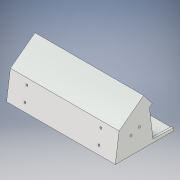
# Autodesk Inventor part: plowV4
Saved by Autodesk Inventor 2019 (Build 230136000, 136)
## iProperties
Created: 2019-04-14
Part Number: plowV4
Material: Generic
Document SubType Name: Modeling
Designer: Tesler
Density: 1 g/cm^3
Appearance: Default
Author: Tesler
Autodesk Inventor part; units mm, degrees
ref_plane "YZ Plane" through (0, 0, 0) normal (1, 0, 0) x (0, 1, 0)
ref_plane "XZ Plane" through (0, 0, 0) normal (0, 1, 0) x (-1, 0, 0)
sketch "Sketch1" plane through (0, 0, 0) normal (1, 0, 0) x (0, 1, 0)
  line L0 (0, 0) -> (0, -85)
  line L1 (0, 0) -> (39.6107, -5.5669)
  line L2 (0, 0) -> (40, 0) construction
  line L3 (39.6107, -5.5669) -> (66.6924, -41.5055)
  line L4 (66.6924, -41.5055) -> (49.9211, -54.1436)
  line L5 (49.9211, -54.1436) -> (47.2715, -49.9034)
  line L6 (0, -85) -> (4, -85)
  line L7 (5, -55) -> (4, -85)
  line L8 (5, -55) -> (47.2715, -49.9034)
  dimension "d0" = 85
  dimension "d1" = 40
  dimension "d2" = 8
  dimension "d3" = 45
  dimension "d4" = 135
  dimension "d5" = 21
  dimension "d6" = 5
  dimension "d7" = 85
  dimension "d12" = 4
  dimension "d13" = 5
  dimension "d50" = 30
  constraints: 18 end point, 2 horizontal, 1 equal length, 1 perpendicular, 1 vertical
  measures "d0" distance of L0.start L0.end
  measures "d1" distance of L0.start L1.end
  measures "d2" angle of L1 L2
  measures "d3" distance of L1.end L3.end
  measures "d4" angle of L1 L3
  measures "d5" distance of L3.end L4.end
  measures "d6" distance of L4.end L5.end
  measures "d7" angle of L4 L5
  measures "d12" distance of L0.end L6.end
  measures "d13" distance from line of L7.start L0
  measures "d50" vertical distance of L7.start L6.end
extrude "Extrusion1" add sketch "Sketch1" along normal blind 3
sketch "Sketch2" plane through (3, 0, 0) normal (1, 0, 0) x (0, 0, -1)
  line L0 (0, 0) -> (85, 0) projected
  line L1 (85, 0) -> (85, 4) projected
  line L2 (85, 4) -> (55, 5) projected
  line L3 (49.9034, 47.2715) -> (54.1436, 49.9211) projected
  line L4 (54.1436, 49.9211) -> (41.5055, 66.6924) projected
  line L5 (41.5055, 66.6924) -> (5.5669, 39.6107) projected
  line L6 (5.5669, 39.6107) -> (0, 0) projected
  line L7 (49.9034, 47.2715) -> (54.1436, 49.9211) projected
  line L8 (51.1436, 48.0464) -> (40.9151, 62.491)
  line L9 (41.5055, 66.6924) -> (5.5669, 39.6107) projected
  line L10 (54.1436, 49.9211) -> (41.5055, 66.6924) projected
  line L11 (40.9151, 62.491) -> (8.3648, 37.9627)
  line L12 (8.3648, 37.9627) -> (3, 3)
  line L13 (5.5669, 39.6107) -> (0, 0) projected
  line L14 (3, 3) -> (85, 3)
  line L15 (85, 0) -> (85, 4) projected
  line L16 (85, 3) -> (85, 0)
  line L17 (0, 0) -> (85, 0) projected
  line L18 (85, 0) -> (0, 0)
  line L19 (0, 0) -> (5.5669, 39.6107)
  line L20 (5.5669, 39.6107) -> (41.5055, 66.6924)
  line L21 (41.5055, 66.6924) -> (54.1436, 49.9211)
  line L22 (54.1436, 49.9211) -> (51.1436, 48.0464)
  line L23 (55, 5) -> (49.9034, 47.2715) projected
  dimension "d14" = 3
  dimension "d15" = 3
  dimension "d16" = 3
  dimension "d17" = 3
  dimension "d18" = 3
  dimension "d21" = 3
  dimension "d22" = 3
  dimension "d23" = 3
  constraints: 20 end point, 4 collinear, 2 point on line, 1 other
  measures "d14" distance from line of L4 L8.end
  measures "d15" horizontal distance of L3.end L8.start
  measures "d16" distance from line of L8.end L5
  measures "d17" distance from line of L5 L11.end
  measures "d18" distance from line of L11.end L6
  measures "d21" distance from line of L0 L14.end
  measures "d22" distance from line of L12.end L0
  measures "d23" horizontal distance of L17.start L12.end
extrude "Extrusion2" add sketch "Sketch2" along normal blind 153 contours L6 L5 L4 L3 L8 L11 L12 L14 L1 L0
ref_plane "Work Plane1" through (79.5, 0, 0) normal (1, 0, 0) x (0, 0, -1)
mirror "Mirror1" about plane through (79.5, 0, 0) normal (1, 0, 0) of "Extrusion1"
sketch "Sketch3" plane through (159, 0, -85) normal (1, 0, 0) x (0, 0, -1)
  line L0 (-85, 0) -> (0, 0) projected
  line L1 (-79.4331, 39.6107) -> (-85, 0) projected
  circle A0 centre (-62.193, 25.4) radius 1.5
  circle A1 centre (-49.984, 30) radius 1.5
  dimension "d28" = 25.4
  dimension "d29" = 30
  dimension "d31" = 19.05
  dimension "d32" = 30.5
  dimension "d33" = 3
  dimension "d34" = 3
  constraints: 2 centre point, 2 coincident
  measures "d28" distance from line of L0 point (-62.193, 25.4)
  measures "d29" distance from line of L0 point (-49.984, 30)
  measures "d31" distance from line of point (-62.193, 25.4) L1
  measures "d32" distance from line of point (-49.984, 30) L1
  measures "d33" diameter of A0
  measures "d34" diameter of A1
extrude "Extrusion3" cut sketch "Sketch3" against normal blind 200
sketch "Sketch4" plane through (0, 0, 0) normal (0, 0.1392, 0.9903) x (1, 0, 0)
  line L0 (0, 0) -> (159, 0) projected
  line L1 (0, 40) -> (0, 0) projected
  line L2 (159, 40) -> (159, 0) projected
  circle A0 centre (25.4, 31.75) radius 1.5
  circle A1 centre (25.4, 11.1125) radius 1.5
  circle A2 centre (133.6, 31.75) radius 1.5
  circle A3 centre (133.6, 11.1125) radius 1.5
  dimension "d37" = 11.1125
  dimension "d38" = 31.75
  dimension "d39" = 25.4
  dimension "d40" = 31.75
  dimension "d41" = 11.1125
  dimension "d42" = 25.4
  dimension "d43" = 3
  dimension "d44" = 3
  dimension "d45" = 3
  dimension "d46" = 3
  constraints: 4 centre point, 4 coincident, 2 vertical alignment
  measures "d37" distance from line of L0 point (25.4, 11.113)
  measures "d38" distance from line of L0 point (25.4, 31.75)
  measures "d39" distance from line of L1 point (25.4, 31.75)
  measures "d40" distance from line of L0 point (133.6, 31.75)
  measures "d41" distance from line of L0 point (133.6, 11.113)
  measures "d42" distance from line of L2 point (133.6, 31.75)
  measures "d43" diameter of A0
  measures "d44" diameter of A1
  measures "d45" diameter of A2
  measures "d46" diameter of A3
extrude "Extrusion4" cut sketch "Sketch4" against normal blind 10
equation "\"d40\" = d38"
equation "\"d41\" = d37"
equation "\"d42\" = d39"
body "Solid1"
